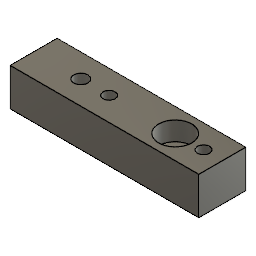
Endstop X&Y Holder (Autodesk Fusion 360 design; units mm, degrees)
Autodesk Fusion 360 part; units mm, degrees
note: some values were not read from the file. Set by a fixed rule: which sketch regions a step uses.
sketch "Skizze1" plane through (0, 0, 0) normal (0, 1, 0) x (1, 0, 0)
  line L0 (0, 0) -> (40, 0)
  line L1 (40, 0) -> (40, -5)
  line L2 (40, -5) -> (40, -10)
  line L3 (40, -10) -> (0, -10)
  line L4 (0, -10) -> (0, 0)
  constraint coincident L0.start L4.end
  constraint horizontal L0
  constraint perpendicular L0 L1
  constraint parallel L1 L2
  constraint perpendicular L2 L3
  constraint perpendicular L3 L4
extrude "Extrusion1" add sketch "Skizze1" along normal blind 8
sketch "Skizze2" plane through (0, 8, 0) normal (0, 1, 0) x (-1, 0, 0)
  line L0 (0, 10) -> (-40, 10)
  line L1 (-40, 10) -> (-40, 0)
  line L2 (-40, 0) -> (0, 0)
  line L3 (0, 0) -> (0, 10)
  circle A0 centre (-10, 5) radius 1.5
  line L4 (-40, 0) -> (-40, 5)
  circle A1 centre (-36, 5) radius 1.275
  circle A2 centre (-16, 5) radius 1.275
  line L5 (-10, 5) -> (-30, 5)
  circle A3 centre (-30, 5) radius 1.5
  circle A4 centre (-30, 5) radius 3.5
  dimension "d3" = 3
  dimension "d4" = 2.55
  dimension "d5" = 2.55
  dimension "d6" = 3
  dimension "d7" = 7
  constraint coincident L1.end L2.start
  constraint midpoint L1 L4.end
  constraint coincident A0.centre L5.start
  constraint horizontal L5
  constraint coincident L5.end A3.centre
  measures "d3" diameter of A0
  measures "d4" diameter of A1
  measures "d5" diameter of A2
  measures "d6" diameter of A3
  measures "d7" diameter of A4
extrude "Extrusion2" cut sketch "Skizze2" against normal blind 20 contours A0 | A3
extrude "Extrusion3" cut sketch "Skizze2" against normal blind 5 contours A2 L5 | A2 L5
extrude "Extrusion4" cut sketch "Skizze2" against normal blind 5 contours A1
extrude "Extrusion5" cut sketch "Skizze2" against normal blind 4 contours A4
